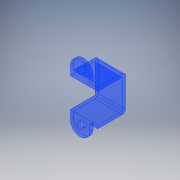
# Autodesk Inventor part: Wheel Mount
Saved by Autodesk Inventor 2017 (Build 210142000, 142)
## iProperties
Created: 2018-02-23
Part Number: Wheel Mount
Material: Aluminum 6061
Document SubType Name: Modeling
Designer: bradl
Density: 2.7 g/cm^3
Appearance: Aluminum - Flat
Author: bradl
Autodesk Inventor part; units mm, degrees
ref_plane "YZ Plane" through (0, 0, 0) normal (1, 0, 0) x (0, 1, 0)
ref_plane "XZ Plane" through (0, 0, 0) normal (0, 1, 0) x (-1, 0, 0)
ref_plane "XY Plane" through (0, 0, 0) normal (0, 0, 1) x (1, 0, 0)
sketch "Sketch1" plane through (0, 0, 0) normal (0, 0, 1) x (1, 0, 0)
  circle A0 centre (0, 0) radius 2 projected
  circle A1 centre (0, 0) radius 9.1281
  point P0 (0, 0)
  dimension "d0" = 18.2563
  constraints: 1 centre point, 1 coincident
  measures "d0" diameter of A1
extrude "Extrusion1" add sketch "Sketch1" against normal blind 4.7625
sketch "Sketch2" plane through (0, 0, 0) normal (0, 0, 1) x (1, 0, 0)
  line L0 (1.118, -1) -> (-1.118, -1) projected
  circle A0 centre (0, 0) radius 2 projected
  circle A1 centre (0, 0) radius 9.1281 projected
  line L1 (0, 0) -> (0, -6.858)
  circle A2 centre (0, -6.858) radius 1.27
  circle A3 centre (6.858, 0) radius 1.27
  circle A4 centre (0, 6.858) radius 1.27
  circle A5 centre (-6.858, 0) radius 1.27
  point P0 (0, 0)
  dimension "d3" = 6.858
  dimension "d4" = 2.54
  dimension "d7" = 360
  constraints: 4 centre point, 2 end point, 1 coincident, 1 vertical, 9 other
  measures "d3" distance of L1.start L1.end
  measures "d4" diameter of A2
extrude "Extrusion2" cut sketch "Sketch2" against normal blind 6.35 contours A2 | A3 | A4 | A5
body "Solid1"
